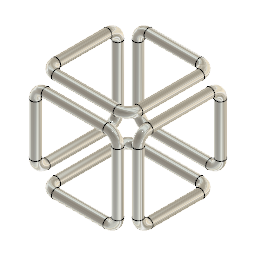
Cubic Pipe v1 (Autodesk Fusion 360 design; units mm, degrees)
Autodesk Fusion 360 part; units mm, degrees
box "BoxPrimitive1" add length 10 width 10 height 10 placed x (0, 1, 0) y (-1, 0, 0) z (0, 0, 1) at (10, 0, 0) makes body 1
sketch "Sketch3" plane through (0, 0, 0) normal (0, -1, 0) x (1, 0, 0)
  line L0 (0, 10) -> (0, 0)
  line L1 (0, 0) -> (10, 0)
  line L2 (10, 0) -> (10, 10)
  line L3 (10, 10) -> (0, 10)
  line L4 (0, 0) -> (2, 0) construction
  line L5 (2, 0) -> (2, 2) construction
  line L6 (2, 2) -> (0, 2) construction
  line L7 (0, 2) -> (0, 0) construction
  line L8 (3, 1) -> (8, 1)
  line L9 (9, 2) -> (9, 8)
  line L10 (8, 9) -> (2, 9)
  line L11 (1, 8) -> (1, 3)
  line L12 (1, 2, -1) -> (1, 2, -7)
  line L13 (1, 3, -8) -> (1, 9, -8)
  line L14 (1, 10, -7) -> (1, 10, -2)
  line L15 (2, 10, -1) -> (8, 10, -1)
  line L16 (9, 10, -2) -> (9, 10, -8)
  line L17 (8, 10, -9) -> (3, 10, -9)
  line L18 (2, 9, -9) -> (2, 3, -9)
  line L19 (3, 2, -9) -> (9, 2, -9)
  line L20 (10, 3, -9) -> (10, 8, -9)
  line L21 (10, 9, -8) -> (10, 9, -2)
  line L22 (10, 8, -1) -> (10, 2, -1)
  line L23 (10, 1, -2) -> (10, 1, -7)
  line L24 (9, 1, -8) -> (3, 1, -8)
  line L25 (2, 1, -7) -> (2, 1, -1)
  arc A0 (2, 9) -> (1, 8) centre (2, 8) ccw
  arc A1 through (2, 10, -1) (1.292893, 10, -1.292893) (1, 10, -2)
  arc A2 (9, 8) -> (8, 9) centre (8, 8) ccw
  arc A3 through (10, 8, -1) (10, 8.707107, -1.292893) (10, 9, -2)
  arc A4 through (9, 10, -2) (8.707107, 10, -1.292893) (8, 10, -1)
  arc A5 through (1, 10, -7) (1, 9.707107, -7.707107) (1, 9, -8)
  arc A6 through (3, 10, -9) (2.292893, 9.707107, -9) (2, 9, -9)
  arc A7 through (10, 9, -8) (10, 8.707107, -8.707107) (10, 8, -9)
  arc A8 through (8, 10, -9) (8.707107, 10, -8.707107) (9, 10, -8)
  arc A9 through (9, 2, -9) (9.707107, 2.292893, -9) (10, 3, -9)
  arc A10 through (2, 3, -9) (2.292893, 2.292893, -9) (3, 2, -9)
  arc A11 through (2, 1, -7) (2.292893, 1, -7.707107) (3, 1, -8)
  arc A12 through (2, 1, -1) (2.292893, 1, -0.292893) (3, 1, 0)
  arc A13 through (1, 2, -1) (1, 2.292893, -0.292893) (1, 3, 0)
  arc A14 through (1, 3, -8) (1, 2.292893, -7.707107) (1, 2, -7)
  arc A15 (8, 1) -> (9, 2) centre (8, 2) ccw
  arc A16 through (10, 1, -2) (10, 1.292893, -1.292893) (10, 2, -1)
  arc A17 through (9, 1, -8) (9.707107, 1, -7.707107) (10, 1, -7)
  point P0 (2, 1)
  point P1 (9, 1)
  point P2 (9, 9)
  point P3 (1, 9)
  point P4 (1, 2)
  point P5 (1, 2)
  point P6 (1, 10)
  point P7 (1, 10)
  point P8 (9, 10)
  point P9 (9, 10)
  point P10 (2, 10)
  point P11 (2, 2)
  point P12 (10, 2)
  point P13 (10, 9)
  point P14 (10, 9)
  point P15 (10, 1)
  point P16 (10, 1)
  point P17 (2, 1)
  dimension "d6" = 2
  dimension "d7" = 2
  dimension "d8" = 7
  dimension "d9" = 90
  dimension "d10" = 8
  dimension "d11" = 8
  dimension "d15" = 8
  dimension "d16" = 8
  dimension "d17" = 7
  dimension "d18" = 8
  dimension "d19" = 8
  dimension "d20" = 7
  dimension "d21" = 8
  dimension "d22" = 8
  dimension "d23" = 7
  dimension "d24" = 8
  dimension "d25" = 8
  dimension "d26" = 7
  dimension "d27" = 8
  dimension "d32" = 1
  constraint horizontal L4
  constraint vertical L5
  constraint horizontal L6
  constraint vertical L7
  constraint coincident L0.end L1.start
  constraint midpoint L5 P17
  constraint perpendicular L5 L8
  constraint perpendicular L5 L10
  constraint midpoint L6 P5
  constraint coincident P3 L10
  constraint coincident P3 L11
  constraint tangent L10 A0
  constraint tangent L11 A0
  constraint coincident P2 L9
  constraint coincident P2 L10
  constraint tangent L9 A2
  constraint tangent L10 A2
  constraint equal A0 A2
  constraint coincident P17 L8
  constraint coincident P5 L11
  constraint coincident P1 L8
  constraint coincident P1 L9
  constraint tangent L8 A15
  constraint tangent L9 A15
  constraint equal A0 A15
  measures "d6" distance of L0.end L4.end
  measures "d7" distance of L0.end L6.end
  measures "d8" distance of P17 P1
  measures "d9" angle of L8 L9
  measures "d10" distance of P1 P2
  measures "d11" distance of P2 P3
  measures "d15" distance of P5 P4
  measures "d16" distance of P5 P7
  measures "d17" distance of P7 P6
  measures "d18" distance of P7 P9
  measures "d19" distance of P9 P8
  measures "d20" distance of P9 P10
  measures "d21" distance of P10 P11
  measures "d22" distance of P11 P12
  measures "d23" distance of P12 P14
  measures "d24" distance of P14 P13
  measures "d25" distance of P14 P16
  measures "d26" distance of P16 P15
  measures "d27" distance of P16 P17
  measures "d32" radius of A0
pipe "Pipe1" add diameter 0.9 path "Sketch3" along A4 L15 A1 L14 A5 L13 A14 L12 A13 L11 A0 L10 A2 L9 A15 L8 A12 L25 A11 L24 A17 L23 A16 L22 A3 L21 A7 L20 A9 L19 A10 L18 A6 L17 A8 L16 separate body makes body 2
hidden bodies 1
